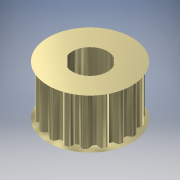
# Autodesk Inventor part: Spur Gear1
Saved by Autodesk Inventor 2016 (Build 200138000, 138)
## iProperties
Created: 2016-11-30
Part Number: Spur Gear1
Material: Steel
Document SubType Name: Modeling
Designer: User
Categories: <?xml version="1.0" encoding="UTF-16"?> <MemberInstance><Categories><FamilyTemplate><FamilyTemplateParameter ValueType="xs:double" Id="1" ObjectReferenceKey="da_z" ObjectType="kUserParameterObject"/><FamilyTemplateParameter ValueType="xs:double" Id="2" ObjectReferenceKey="da_b" ObjectType="kUserParameterObject"/><FamilyTemplateParameter ValueType="xs:double" Id="3" ObjectReferenceKey="da_beta" ObjectType="kUserParameterObject"/><FamilyTemplateParameter ValueType="xs:double" Id="4" ObjectReferenceKey="da_da" ObjectType="kUserParameterObject"/><FamilyTemplateParameter ValueType="xs:double" Id="5" ObjectReferenceKey="da_aw" ObjectType="kUserParameterObject"/><FamilyTemplateParameter ValueType="xs:string" Id="6" ObjectReferenceKey="EAIAABAAAACIAQAAAAAAAIAAAAAAAAAA" ObjectType="83910656" SubObjectId="SurfaceGeometry"/></FamilyTemplate><ParamToTemplateMap><ParamToTemplate CategoryParameter="//CategoryParameter[@InternalName='046C89C9-8512-4d59-83FE-43B91F4F132A']" TemplateParameter="1"/><ParamToTemplate CategoryParameter="//CategoryParameter[@InternalName='2552DF32-E462-4b46-AEBF-C6C7768E72AC']" TemplateParameter="2"/><ParamToTemplate CategoryParameter="//CategoryParameter[@InternalName='C9EE641D-15FC-4fae-A226-E94C4372FDD7']" TemplateParameter="3"/><ParamToTemplate><ParamToTemplate CategoryParameter="//CategoryParameter[@InternalName='00B6519A-459B-49c7-AD84-2E56D39A5744']" ConstantValue="0.000000"/></ParamToTemplate><ParamToTemplate><ParamToTemplate CategoryParameter="//CategoryParameter[@InternalName='04B31F0E-C7A6-4894-AA32-9629BEFACF47']" ConstantValue="1.000000"/></ParamToTemplate><ParamToTemplate><ParamToTemplate CategoryParameter="//CategoryParameter[@InternalName='43CBEC2E-7847-49e7-A936-2F7889FCB2D9']" ConstantValue="0.250000"/></ParamToTemplate><ParamToTemplate><ParamToTemplate CategoryParameter="//CategoryParameter[@InternalName='B1EFC894-105D-4ebd-86BF-FA20ED196853']" ConstantValue="0.350000"/></ParamToTemplate><ParamToTemplate><ParamToTemplate CategoryParameter="//CategoryParameter[@InternalName='51175063-3D10-4879-93E8-6246FE8B403D']" ConstantValue="2060000000.000000"/></ParamToTemplate><ParamToTemplate><ParamToTemplate CategoryParameter="//CategoryParameter[@InternalName='A3A52E27-4454-46a9-B0BD-C932399B70AF']" ConstantValue="0.300000"/></ParamToTemplate><ParamToTemplate><ParamToTemplate CategoryParameter="//CategoryParameter[@InternalName='91B76062-C214-41d9-B1B9-14D2AB99603D']" ConstantValue="0.250000"/></ParamToTemplate><ParamToTemplate><ParamToTemplate CategoryParameter="//CategoryParameter[@InternalName='374E806E-8B8A-4dda-A9AA-1039D6500AD2']" ConstantValue="4.000000"/></ParamToTemplate><ParamToTemplate><ParamToTemplate CategoryParameter="//CategoryParameter[@InternalName='2D373A89-B862-43d6-8D0B-0CBF12AB9F6C']" ConstantValue="0.349066"/></ParamToTemplate><ParamToTemplate CategoryParameter="//CategoryParameter[@InternalName='37777632-D6A2-4fac-9D53-DB8ACD95C989']" TemplateParameter="4"/><ParamToTemplate CategoryParameter="//CategoryParameter[@InternalName='FD1017F1-B727-4f7e-9707-0F86F1FF9423']" TemplateParameter="5"/><ParamToTemplate><ParamToTemplate CategoryParameter="//CategoryParameter[@InternalName='9E1B4470-B2D3-4ff1-B813-535BB4CDF51A']" ConstantValue="3520000.000000"/></ParamToTemplate><ParamToTemplate><ParamToTemplate CategoryParameter="//CategoryParameter[@InternalName='F8452263-BFF6-458c-9FB1-07C4B99E95CD']" ConstantValue="11400000.000000"/></ParamToTemplate><ParamToTemplate><ParamToTemplate CategoryParameter="//CategoryParameter[@InternalName='3E3BB259-FD49-497f-8171-6EBC954A3479']" ConstantValue="2.000000"/></ParamToTemplate><ParamToTemplate CategoryParameter="//CategoryParameter[@InternalName='27C3BAF2-7550-4e4b-AE2C-0DB134B7D9B7']" TemplateParameter="6"/></ParamToTemplateMap><Category DisplayName="Gear" InternalName="DC85795E-93AB-48d5-8EEE-5A27447B64BD" Mnemonic="Gear"><CategoryParameter DisplayName="z" InternalName="046C89C9-8512-4d59-83FE-43B91F4F132A" Mnemonic="z"/><CategoryParameter DisplayName="b" InternalName="2552DF32-E462-4b46-AEBF-C6C7768E72AC" Mnemonic="b"/><CategoryParameter DisplayName="||b|" InternalName="C9EE641D-15FC-4fae-A226-E94C4372FDD7" Mnemonic="beta"/><CategoryParameter DisplayName="x" InternalName="00B6519A-459B-49c7-AD84-2E56D39A5744" Mnemonic="x"/><CategoryParameter DisplayName="a*" InternalName="04B31F0E-C7A6-4894-AA32-9629BEFACF47" Mnemonic="a"/><CategoryParameter DisplayName="c*" InternalName="43CBEC2E-7847-49e7-A936-2F7889FCB2D9" Mnemonic="c"/><CategoryParameter DisplayName="r|.f|*" InternalName="B1EFC894-105D-4ebd-86BF-FA20ED196853" Mnemonic="rf"/><CategoryParameter DisplayName="E" InternalName="51175063-3D10-4879-93E8-6246FE8B403D" Mnemonic="E"/><CategoryParameter DisplayName="||m|" InternalName="A3A52E27-4454-46a9-B0BD-C932399B70AF" Mnemonic="mi"/><Category DisplayName="SpurGear" InternalName="26C5A22E-A91E-4dfd-A3B3-23CCAFAE1764" Mnemonic="SpurGear"><CategoryParameter DisplayName="m" InternalName="91B76062-C214-41d9-B1B9-14D2AB99603D" Mnemonic="m"/><CategoryParameter DisplayName="P" InternalName="374E806E-8B8A-4dda-A9AA-1039D6500AD2" Mnemonic="PP"/><CategoryParameter DisplayName="||a|" InternalName="2D373A89-B862-43d6-8D0B-0CBF12AB9F6C" Mnemonic="alpha"/><CategoryParameter DisplayName="d|.a|" InternalName="37777632-D6A2-4fac-9D53-DB8ACD95C989" Mnemonic="da"/><CategoryParameter DisplayName="a|.w|" InternalName="FD1017F1-B727-4f7e-9707-0F86F1FF9423" Mnemonic="aw"/><CategoryParameter DisplayName="||s||.Flim|" InternalName="9E1B4470-B2D3-4ff1-B813-535BB4CDF51A" Mnemonic="sFlim"/><CategoryParameter DisplayName="||s||.Hlim|" InternalName="F8452263-BFF6-458c-9FB1-07C4B99E95CD" Mnemonic="sHlim"/><CategoryParameter DisplayName="type" InternalName="3E3BB259-FD49-497f-8171-6EBC954A3479" Mnemonic="type"/><CategoryParameter DisplayName="PitchDiameter" InternalName="27C3BAF2-7550-4e4b-AE2C-0DB134B7D9B7" Mnemonic="IDS_PITCHDIAM"/></Category></Category></Categories></MemberInstance>
Density: 1 g/cm^3
Appearance: Gold - Metal
CustomPartVersion: 1
Author: User
Autodesk Inventor part; units mm, degrees
sketch "Sketch1" plane through (0, 0, 0) normal (0, 0, 1) x (1, 0, 0)
  circle A0 centre (0, 0) radius 5.5
  dimension "d0" = 11
  constraints: 1 centre point
  measures "d0" diameter of A0
extrude "Extrusion1" add sketch "Sketch1" along normal blind 7
ref_plane "Work Plane2" through (0, 0, 3.5) normal (0, 0, 1) x (1, 0, 0)
sketch "Sketch2" plane through (0, 0, 0) normal (0, 0, -1) x (-1, 0, 0)
  circle A0 centre (0, 0) radius 5.5 projected
  circle A1 centre (0, 0) radius 22.8571
  dimension "d3" = 45.7143
  constraints: 1 centre point, 1 coincident
  measures "d3" diameter of A1
feature "Pitch Diameter" [suppressed]
ref_plane "Work Plane8" through (0, 0, 0) normal (0.9848078, 0.1736482, 0) x (0, 0, 1)
ref_plane "Work Plane9" through (0, 0, 0) normal (1, 0, 0) x (0, 1, 0)
spur gear teeth "Spur Gear" teeth 18 pitch diameter 8 tip diameter 11 root diameter 10 face width 7 start plane through (0, 0, 0) normal (0, 0, -1) x (-1, 0, 0)
sketch "Sketch3" plane through (0, 0, 7) normal (0, 0, 1) x (1, 0, 0)
  arc A0 (-0.6526, 4.9572) -> (-1.0822, 4.8815) centre (0, 0) ccw projected
  arc A1 (-0.2399, 5.4948) -> (-0.6526, 4.9572) centre (1.0466, 4.0798) ccw projected
  arc A2 (0.2399, 5.4948) -> (-0.2399, 5.4948) centre (0, 0) ccw projected
  arc A3 (0.6526, 4.9572) -> (0.2399, 5.4948) centre (-1.0466, 4.0798) ccw projected
  arc A4 (1.0822, 4.8815) -> (0.6526, 4.9572) centre (0, 0) ccw projected
  arc A5 (1.6539, 5.2454) -> (1.0822, 4.8815) centre (2.3788, 3.4758) ccw projected
  arc A6 (2.1048, 5.0813) -> (1.6539, 5.2454) centre (0, 0) ccw projected
  arc A7 (2.3087, 4.4351) -> (2.1048, 5.0813) centre (0.4119, 4.1917) ccw projected
  arc A8 (2.6865, 4.217) -> (2.3087, 4.4351) centre (0, 0) ccw projected
  arc A9 (3.3482, 4.3634) -> (2.6865, 4.217) centre (3.4242, 2.4526) ccw projected
  arc A10 (3.7157, 4.055) -> (3.3482, 4.3634) centre (0, 0) ccw projected
  arc A11 (3.6864, 3.378) -> (3.7157, 4.055) centre (1.8207, 3.798) ccw projected
  arc A12 (3.9668, 3.0438) -> (3.6864, 3.378) centre (0, 0) ccw projected
  arc A13 (4.6387, 2.9551) -> (3.9668, 3.0438) centre (4.0565, 1.1336) ccw projected
  arc A14 (4.8786, 2.5396) -> (4.6387, 2.9551) centre (0, 0) ccw projected
  arc A15 (4.6194, 1.9134) -> (4.8786, 2.5396) centre (3.0099, 2.9462) ccw projected
  arc A16 (4.7686, 1.5035) -> (4.6194, 1.9134) centre (0, 0) ccw projected
  arc A17 (5.3696, 1.1904) -> (4.7686, 1.5035) centre (4.1996, -0.3222) ccw projected
  arc A18 (5.4529, 0.7179) -> (5.3696, 1.1904) centre (0, 0) ccw projected
  arc A19 (4.9952, 0.2181) -> (5.4529, 0.7179) centre (3.8361, 1.7391) ccw projected
  arc A20 (4.9952, -0.2181) -> (4.9952, 0.2181) centre (0, 0) ccw projected
  arc A21 (5.4529, -0.7179) -> (4.9952, -0.2181) centre (3.8361, -1.7391) ccw projected
  arc A22 (5.3696, -1.1904) -> (5.4529, -0.7179) centre (0, 0) ccw projected
  arc A23 (4.7686, -1.5035) -> (5.3696, -1.1904) centre (4.1996, 0.3222) ccw projected
  arc A24 (4.6194, -1.9134) -> (4.7686, -1.5035) centre (0, 0) ccw projected
  arc A25 (4.8786, -2.5396) -> (4.6194, -1.9134) centre (3.0099, -2.9462) ccw projected
  arc A26 (4.6387, -2.9551) -> (4.8786, -2.5396) centre (0, 0) ccw projected
  arc A27 (3.9668, -3.0438) -> (4.6387, -2.9551) centre (4.0565, -1.1336) ccw projected
  arc A28 (3.6864, -3.378) -> (3.9668, -3.0438) centre (0, 0) ccw projected
  arc A29 (3.7157, -4.055) -> (3.6864, -3.378) centre (1.8207, -3.798) ccw projected
  arc A30 (3.3482, -4.3634) -> (3.7157, -4.055) centre (0, 0) ccw projected
  arc A31 (2.6865, -4.217) -> (3.3482, -4.3634) centre (3.4242, -2.4526) ccw projected
  arc A32 (2.3087, -4.4351) -> (2.6865, -4.217) centre (0, 0) ccw projected
  arc A33 (2.1048, -5.0813) -> (2.3087, -4.4351) centre (0.4119, -4.1917) ccw projected
  arc A34 (1.6539, -5.2454) -> (2.1048, -5.0813) centre (0, 0) ccw projected
  arc A35 (1.0822, -4.8815) -> (1.6539, -5.2454) centre (2.3788, -3.4758) ccw projected
  arc A36 (0.6526, -4.9572) -> (1.0822, -4.8815) centre (0, 0) ccw projected
  arc A37 (0.2399, -5.4948) -> (0.6526, -4.9572) centre (-1.0466, -4.0798) ccw projected
  arc A38 (-0.2399, -5.4948) -> (0.2399, -5.4948) centre (0, 0) ccw projected
  arc A39 (-0.6526, -4.9572) -> (-0.2399, -5.4948) centre (1.0466, -4.0798) ccw projected
  arc A40 (-1.0822, -4.8815) -> (-0.6526, -4.9572) centre (0, 0) ccw projected
  arc A41 (-1.6539, -5.2454) -> (-1.0822, -4.8815) centre (-2.3788, -3.4758) ccw projected
  arc A42 (-2.1048, -5.0813) -> (-1.6539, -5.2454) centre (0, 0) ccw projected
  arc A43 (-2.3087, -4.4351) -> (-2.1048, -5.0813) centre (-0.4119, -4.1917) ccw projected
  arc A44 (-2.6865, -4.217) -> (-2.3087, -4.4351) centre (0, 0) ccw projected
  arc A45 (-3.3482, -4.3634) -> (-2.6865, -4.217) centre (-3.4242, -2.4526) ccw projected
  arc A46 (-3.7157, -4.055) -> (-3.3482, -4.3634) centre (0, 0) ccw projected
  arc A47 (-3.6864, -3.378) -> (-3.7157, -4.055) centre (-1.8207, -3.798) ccw projected
  arc A48 (-3.9668, -3.0438) -> (-3.6864, -3.378) centre (0, 0) ccw projected
  arc A49 (-4.6387, -2.9551) -> (-3.9668, -3.0438) centre (-4.0565, -1.1336) ccw projected
  arc A50 (-4.8786, -2.5396) -> (-4.6387, -2.9551) centre (0, 0) ccw projected
  arc A51 (-4.6194, -1.9134) -> (-4.8786, -2.5396) centre (-3.0099, -2.9462) ccw projected
  arc A52 (-4.7686, -1.5035) -> (-4.6194, -1.9134) centre (0, 0) ccw projected
  arc A53 (-5.3696, -1.1904) -> (-4.7686, -1.5035) centre (-4.1996, 0.3222) ccw projected
  arc A54 (-5.4529, -0.7179) -> (-5.3696, -1.1904) centre (0, 0) ccw projected
  arc A55 (-4.9952, -0.2181) -> (-5.4529, -0.7179) centre (-3.8361, -1.7391) ccw projected
  arc A56 (-4.9952, 0.2181) -> (-4.9952, -0.2181) centre (0, 0) ccw projected
  arc A57 (-5.4529, 0.7179) -> (-4.9952, 0.2181) centre (-3.8361, 1.7391) ccw projected
  arc A58 (-5.3696, 1.1904) -> (-5.4529, 0.7179) centre (0, 0) ccw projected
  arc A59 (-4.7686, 1.5035) -> (-5.3696, 1.1904) centre (-4.1996, -0.3222) ccw projected
  arc A60 (-4.6194, 1.9134) -> (-4.7686, 1.5035) centre (0, 0) ccw projected
  arc A61 (-4.8786, 2.5396) -> (-4.6194, 1.9134) centre (-3.0099, 2.9462) ccw projected
  arc A62 (-4.6387, 2.9551) -> (-4.8786, 2.5396) centre (0, 0) ccw projected
  arc A63 (-3.9668, 3.0438) -> (-4.6387, 2.9551) centre (-4.0565, 1.1336) ccw projected
  arc A64 (-3.6864, 3.378) -> (-3.9668, 3.0438) centre (0, 0) ccw projected
  arc A65 (-3.7157, 4.055) -> (-3.6864, 3.378) centre (-1.8207, 3.798) ccw projected
  arc A66 (-3.3482, 4.3634) -> (-3.7157, 4.055) centre (0, 0) ccw projected
  arc A67 (-2.6865, 4.217) -> (-3.3482, 4.3634) centre (-3.4242, 2.4526) ccw projected
  arc A68 (-2.3087, 4.4351) -> (-2.6865, 4.217) centre (0, 0) ccw projected
  arc A69 (-2.1048, 5.0813) -> (-2.3087, 4.4351) centre (-0.4119, 4.1917) ccw projected
  arc A70 (-1.6539, 5.2454) -> (-2.1048, 5.0813) centre (0, 0) ccw projected
  arc A71 (-1.0822, 4.8815) -> (-1.6539, 5.2454) centre (-2.3788, 3.4758) ccw projected
  circle A72 centre (0, 0) radius 2.5
  dimension "d49" = 5
  constraints: 1 centre point, 1 coincident
  measures "d49" diameter of A72
extrude "Extrusion2" cut sketch "Sketch3" against normal through all contours A72
sketch "Sketch4" plane through (0, 0, 0) normal (0, 1, 0) x (-1, 0, 0)
  line L0 (5, 7) -> (5, 0) projected
  line L1 (5, 0) -> (2.5, 0) projected
  line L2 (2.5, 0) -> (2.5, 7) projected
  line L3 (2.5, 7) -> (5, 7) projected
  line L4 (-5, 0) -> (-5, 7) projected
  line L5 (-5, 7) -> (-2.5, 7) projected
  line L6 (-2.5, 7) -> (-2.5, 0) projected
  line L7 (-2.5, 0) -> (-5, 0) projected
  line L8 (0, 0) -> (0, 7)
  line L9 (-0.2399, 7) -> (0.2399, 7) projected
  line L10 (-2.5, 7) -> (-5.9316, 7)
  line L11 (-2.5, 7) -> (-2.5, 0) projected
  arc A0 (-5.9316, 7) -> (-2.5, 6.5) centre (-2.5, 18.5256) ccw
  line L12 (-2.5, 6.5) -> (-8.7939, 6.5) construction
  dimension "d52" = 0.5
  constraints: 6 end point, 2 horizontal, 2 point on circle, 1 centre point, 1 midpoint, 1 point on line, 1 tangent
  measures "d52" distance of L5.end L12.start
revolve "Revolution1" add sketch "Sketch4" angle 360 about axis through (0, 0, 0) along (0, 0, 1) contours A0 L10 L4 | L4 L5 L6 A0
ref_plane "Work Plane11" through (0, 0, 3.5) normal (0, 0, 1) x (1, 0, 0)
mirror "Mirror1" about plane through (0, 0, 3.5) normal (0, 0, 1) of "Revolution1"
equation "\"d0\" = da_da"
equation "\"d1\" = da_b"
equation "\"d3\" = da_dw"
equation "\"d16\" = da_aw"
equation "\"da_da\" = 11"
equation "\"da_b\" = 7"
equation "\"da_dw\" = 45.714286"
equation "\"da_aw\" = 80"
body "Solid1"
body "Srf1"
